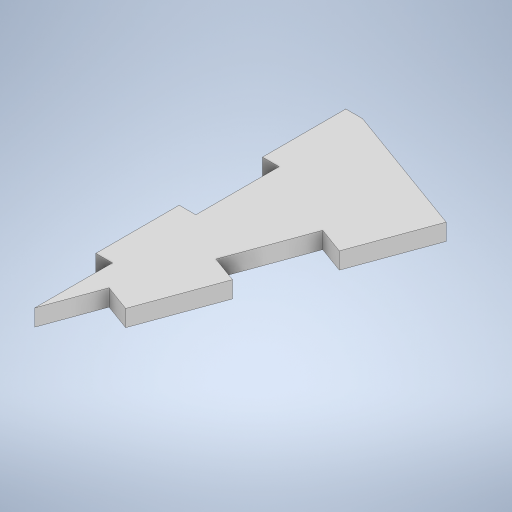
# Autodesk Inventor part: do_sensor_3_3mm
Saved by Autodesk Inventor 2023 (Build 270158000, 158)
## iProperties
Created: 2022-11-21
Part Number: do_sensor_3_3mm
Material: Generic
Document SubType Name: Modeling
Designer: ADMIN
Density: 1 g/cm^3
Appearance: Default
Author: ADMIN
Autodesk Inventor part; units mm, degrees
ref_plane "YZ Plane" through (0, 0, 0) normal (1, 0, 0) x (0, 1, 0)
ref_plane "XZ Plane" through (0, 0, 0) normal (0, 1, 0) x (-1, 0, 0)
ref_plane "XY Plane" through (0, 0, 0) normal (0, 0, 1) x (1, 0, 0)
sketch "Sketch1" plane through (0, 0, 0) normal (0, 1, 0) x (-1, 0, 0)
  line L0 (-13.5, 16) -> (-10.5, 16)
  line L1 (-22.2016, 21.0925) -> (-25.0207, 22.1185)
  line L2 (-10.5, 31) -> (-13.5, 31)
  line L3 (-10.5, 16) -> (-10.5, 31)
  line L4 (-19.8904, 36.2139) -> (-17.0713, 35.1879)
  line L5 (-13.5, 45) -> (-17.0713, 35.1879)
  line L6 (-13.5, 45) -> (-13.5, 31)
  line L7 (-13.5, -14) -> (-32.4622, -7.0983)
  line L8 (-27.3319, 6.9971) -> (-22.2016, 21.0925)
  line L9 (-22.2016, 21.0925) -> (-27.3319, 6.9971)
  line L10 (-13.5, 1) -> (-13.5, 16)
  line L11 (-13.5, 16) -> (-13.5, 1)
  line L12 (-30.151, 8.0231) -> (-27.3319, 6.9971)
  line L13 (-10.5, 1) -> (-13.5, 1)
  line L14 (-13.5, -14) -> (-10.5, -14)
  line L15 (-10.5, -14) -> (-10.5, 1)
  line L16 (-32.4622, -7.0983) -> (-35.2813, -6.0723)
  line L17 (-27.3319, 6.9971) -> (-32.0304, 8.7072)
  line L18 (-32.0304, 8.7072) -> (-37.1607, -5.3882)
  line L19 (-37.1607, -5.3882) -> (-35.2813, -6.0723)
  line L20 (-25.0207, 22.1185) -> (-26.9001, 22.8026)
  line L21 (-26.9001, 22.8026) -> (-21.7698, 36.898)
  line L22 (-21.7698, 36.898) -> (-19.8904, 36.2139)
  point P0 (0, 0)
  point P1 (0, 0)
  dimension "d0" = 3
  dimension "d1" = 15
  dimension "d2" = 15
  dimension "d3" = 15
  dimension "d4" = 15
  dimension "d5" = 15
  dimension "d6" = 15
  dimension "d7" = 2.8191
  dimension "d8" = 5
  constraints: 46 end point, 16 perpendicular, 3 point on line, 1 parallel, 1 vertical
  measures "d0" distance of L7.start L15.start
  measures "d1" distance of L15.start L13.start
  measures "d2" distance of L10.start L0.start
  measures "d3" distance of L0.end L3.end
  measures "d4" distance of L16.end L12.start
  measures "d5" distance of L8.start L8.end
  measures "d6" distance of L1.end L4.start
  measures "d7" horizontal distance of L12.start L8.start
  measures "d8" distance of L8.start L17.end
extrude "Extrusion1" add sketch "Sketch1" along normal blind 3
body "Solid1"
